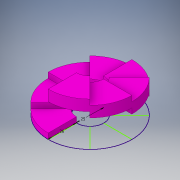
# Autodesk Inventor part: DireccionEscalones
Saved by Autodesk Inventor 2019 (Build 230136000, 136)
## iProperties
Created: 2019-12-22
Part Number: DireccionEscalones
Material: Generic
Document SubType Name: Modeling
Designer: Sergio
Density: 1 g/cm^3
Appearance: Magenta
Author: Sergio
Autodesk Inventor part; units mm, degrees
ref_plane "YZ Plane" through (0, 0, 0) normal (1, 0, 0) x (0, 1, 0)
ref_plane "XZ Plane" through (0, 0, 0) normal (0, 1, 0) x (-1, 0, 0)
ref_plane "XY Plane" through (0, 0, 0) normal (0, 0, 1) x (1, 0, 0)
sketch "Sketch1" plane through (0, 0, 0) normal (0, 1, 0) x (-1, 0, 0)
  circle A0 centre (0, 0) radius 12.5
  circle A1 centre (0, 0) radius 38.5
  line L0 (-8.8388, 8.8388) -> (-27.2236, 27.2236)
  line L1 (8.8388, -8.8388) -> (27.2236, -27.2236)
  line L2 (8.8388, 8.8388) -> (27.2236, 27.2236)
  line L3 (-8.8388, -8.8388) -> (-27.2236, -27.2236)
  line L4 (0, 38.5) -> (0, 12.5)
  line L5 (0, -12.5) -> (0, -38.5)
  line L6 (38.5, 0) -> (12.5, 0)
  line L7 (-12.5, 0) -> (-38.5, 0)
  dimension "d0" = 25
  dimension "d2" = 26
  constraints: 16 end point, 4 perpendicular, 2 coincident, 2 horizontal, 1 point on line, 20 other
sketch "Sketch22" plane through (0, 0, 0) normal (0, 1, 0) x (-1, 0, 0)
  circle A0 centre (0, 0) radius 12.5
  circle A1 centre (0, 0) radius 38.5
  line L0 (-8.8388, 8.8388) -> (-27.2236, 27.2236)
  line L1 (8.8388, -8.8388) -> (27.2236, -27.2236)
  line L2 (8.8388, 8.8388) -> (27.2236, 27.2236)
  line L3 (-8.8388, -8.8388) -> (-27.2236, -27.2236)
  line L4 (0, 38.5) -> (0, 12.5)
  line L5 (0, -12.5) -> (0, -38.5)
  line L6 (38.5, 0) -> (12.5, 0)
  line L7 (-12.5, 0) -> (-38.5, 0)
  circle A2 centre (0, 0) radius 12.5
  circle A3 centre (0, 0) radius 38.5
  line L8 (-8.8388, 8.8388) -> (-27.2236, 27.2236)
  line L9 (8.8388, -8.8388) -> (27.2236, -27.2236)
  line L10 (8.8388, 8.8388) -> (27.2236, 27.2236)
  line L11 (-8.8388, -8.8388) -> (-27.2236, -27.2236)
  line L12 (0, 38.5) -> (0, 12.5)
  line L13 (0, -12.5) -> (0, -38.5)
  line L14 (38.5, 0) -> (12.5, 0)
  line L15 (-12.5, 0) -> (-38.5, 0)
  dimension "d128" = 25
  dimension "d129" = 26
  dimension "d130" = 25
  dimension "d131" = 26
  constraints: 32 end point, 8 perpendicular, 4 coincident, 4 horizontal, 2 point on line, 40 other
sketch "Sketch23" plane through (0, 0, 0) normal (0, 1, 0) x (-1, 0, 0)
  circle A0 centre (0, 0) radius 12.5
  circle A1 centre (0, 0) radius 38.5
  line L0 (-8.8388, 8.8388) -> (-27.2236, 27.2236)
  line L1 (8.8388, -8.8388) -> (27.2236, -27.2236)
  line L2 (8.8388, 8.8388) -> (27.2236, 27.2236)
  line L3 (-8.8388, -8.8388) -> (-27.2236, -27.2236)
  line L4 (0, 38.5) -> (0, 12.5)
  line L5 (0, -12.5) -> (0, -38.5)
  line L6 (38.5, 0) -> (12.5, 0)
  line L7 (-12.5, 0) -> (-38.5, 0)
  dimension "d132" = 25
  dimension "d133" = 26
  constraints: 16 end point, 4 perpendicular, 2 coincident, 2 horizontal, 1 point on line, 20 other
sketch "Sketch24" plane through (0, 0, 0) normal (0, 1, 0) x (-1, 0, 0)
  circle A0 centre (0, 0) radius 12.5
  circle A1 centre (0, 0) radius 38.5
  line L0 (-8.8388, 8.8388) -> (-27.2236, 27.2236)
  line L1 (8.8388, -8.8388) -> (27.2236, -27.2236)
  line L2 (8.8388, 8.8388) -> (27.2236, 27.2236)
  line L3 (-8.8388, -8.8388) -> (-27.2236, -27.2236)
  line L4 (0, 38.5) -> (0, 12.5)
  line L5 (0, -12.5) -> (0, -38.5)
  line L6 (38.5, 0) -> (12.5, 0)
  line L7 (-12.5, 0) -> (-38.5, 0)
  dimension "d134" = 25
  dimension "d135" = 26
  constraints: 16 end point, 4 perpendicular, 2 coincident, 2 horizontal, 1 point on line, 20 other
sketch "Sketch25" plane through (0, 0, 0) normal (0, 1, 0) x (-1, 0, 0)
  circle A0 centre (0, 0) radius 12.5
  circle A1 centre (0, 0) radius 38.5
  line L0 (-8.8388, 8.8388) -> (-27.2236, 27.2236)
  line L1 (8.8388, -8.8388) -> (27.2236, -27.2236)
  line L2 (8.8388, 8.8388) -> (27.2236, 27.2236)
  line L3 (-8.8388, -8.8388) -> (-27.2236, -27.2236)
  line L4 (0, 38.5) -> (0, 12.5)
  line L5 (0, -12.5) -> (0, -38.5)
  line L6 (38.5, 0) -> (12.5, 0)
  line L7 (-12.5, 0) -> (-38.5, 0)
  dimension "d136" = 25
  dimension "d137" = 26
  constraints: 16 end point, 4 perpendicular, 2 coincident, 2 horizontal, 1 point on line, 20 other
sketch "Sketch26" plane through (0, 0, 0) normal (0, 1, 0) x (-1, 0, 0)
  circle A0 centre (0, 0) radius 12.5
  circle A1 centre (0, 0) radius 38.5
  line L0 (-8.8388, 8.8388) -> (-27.2236, 27.2236)
  line L1 (8.8388, -8.8388) -> (27.2236, -27.2236)
  line L2 (8.8388, 8.8388) -> (27.2236, 27.2236)
  line L3 (-8.8388, -8.8388) -> (-27.2236, -27.2236)
  line L4 (0, 38.5) -> (0, 12.5)
  line L5 (0, -12.5) -> (0, -38.5)
  line L6 (38.5, 0) -> (12.5, 0)
  line L7 (-12.5, 0) -> (-38.5, 0)
  dimension "d138" = 25
  dimension "d139" = 26
  constraints: 16 end point, 4 perpendicular, 2 coincident, 2 horizontal, 1 point on line, 20 other
sketch "Sketch27" plane through (0, 0, 0) normal (0, 1, 0) x (-1, 0, 0)
  circle A0 centre (0, 0) radius 12.5
  circle A1 centre (0, 0) radius 38.5
  line L0 (-8.8388, 8.8388) -> (-27.2236, 27.2236)
  line L1 (8.8388, -8.8388) -> (27.2236, -27.2236)
  line L2 (8.8388, 8.8388) -> (27.2236, 27.2236)
  line L3 (-8.8388, -8.8388) -> (-27.2236, -27.2236)
  line L4 (0, 38.5) -> (0, 12.5)
  line L5 (0, -12.5) -> (0, -38.5)
  line L6 (38.5, 0) -> (12.5, 0)
  line L7 (-12.5, 0) -> (-38.5, 0)
  dimension "d140" = 25
  dimension "d141" = 26
  constraints: 16 end point, 4 perpendicular, 2 coincident, 2 horizontal, 1 point on line, 20 other
sketch "Sketch28" plane through (0, 0, 0) normal (0, 1, 0) x (-1, 0, 0)
  circle A0 centre (0, 0) radius 12.5
  circle A1 centre (0, 0) radius 38.5
  line L0 (-8.8388, 8.8388) -> (-27.2236, 27.2236)
  line L1 (8.8388, -8.8388) -> (27.2236, -27.2236)
  line L2 (8.8388, 8.8388) -> (27.2236, 27.2236)
  line L3 (-8.8388, -8.8388) -> (-27.2236, -27.2236)
  line L4 (0, 38.5) -> (0, 12.5)
  line L5 (0, -12.5) -> (0, -38.5)
  line L6 (38.5, 0) -> (12.5, 0)
  line L7 (-12.5, 0) -> (-38.5, 0)
  dimension "d142" = 25
  dimension "d143" = 26
  constraints: 16 end point, 4 perpendicular, 2 coincident, 2 horizontal, 1 point on line, 20 other
extrude "Extrusion20" add sketch "Sketch1" along normal blind 5 contours A0 L4 A1 L2
extrude "Extrusion21" add sketch "Sketch24" along normal blind 10 contours A0 L2 A1 L6
extrude "Extrusion22" add sketch "Sketch22" along normal blind 15 contours L6 A1 L1 A0
extrude "Extrusion23" add sketch "Sketch28" along normal blind 20 contours L1 A1 L5 A0
extrude "Extrusion24" add sketch "Sketch1" along normal blind 25 contours L5 A1 L3 A0
extrude "Extrusion25" add sketch "Sketch27" along normal blind 30 contours L3 A1 L7 A0
extrude "Extrusion26" add sketch "Sketch1" along normal blind 35 contours A0 L7 A1 L0
extrude "Extrusion27" add sketch "Sketch23" along normal blind 40 contours A0 L0 A1 L4
sketch "Sketch29" plane through (0, 0, 0) normal (0, -1, 0) x (1, 0, 0)
  point P0 (0, 0)
extrude "Extrusion28" cut sketch "Sketch26" along normal blind 5 contours L6 A1 L1 A0
extrude "Extrusion29" cut sketch "Sketch25" along normal blind 10 contours L1 A1 L5 A0
extrude "Extrusion30" cut sketch "Sketch1" along normal blind 15 contours L5 A1 L3 A0
extrude "Extrusion31" cut sketch "Sketch1" along normal blind 20 contours L3 A1 L7 A0
extrude "Extrusion32" cut sketch "Sketch1" along normal blind 25 contours A0 L7 A1 L0
extrude "Extrusion33" cut sketch "Sketch1" along normal blind 30 contours A0 L0 A1 L4
body "Solid2"
